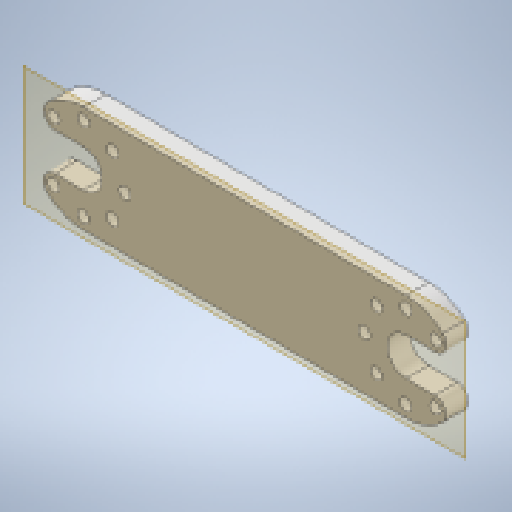
# Autodesk Inventor part: calf
Saved by Autodesk Inventor 2024 (Build 280153000, 153)
## iProperties
Created: 2024-09-17
Part Number: calf
Material: PMMA 플라스틱
Document SubType Name: Modeling
Designer: Eungang
Density: 1.188 g/cm^3
Appearance: 폴리카보네이트 - 선명
Author: Eungang
Autodesk Inventor part; units mm, degrees
ref_plane "YZ Plane" through (0, 0, 0) normal (1, 0, 0) x (0, 1, 0)
ref_plane "XZ Plane" through (0, 0, 0) normal (0, 1, 0) x (-1, 0, 0)
ref_plane "XY Plane" through (0, 0, 0) normal (0, 0, 1) x (1, 0, 0)
ref_plane "작업 평면1" through (0, 0, 0) normal (0, 0, 1) x (1, 0, 0)
sketch "스케치1" plane through (0, 0, 0) normal (0, 0, 1) x (1, 0, 0)
  circle A0 centre (-5.2751, -1.5499) radius 1.55 projected
  circle A1 centre (2.5198, 1.6312) radius 1.55 projected
  circle A2 centre (-16.2175, 9.5075) radius 1.55 projected
  circle A3 centre (-13.0363, 1.7126) radius 1.55 projected
  circle A4 centre (-12.955, 17.2687) radius 1.55 projected
  circle A5 centre (-90.374, -1.1049) radius 1.55 projected
  circle A6 centre (-98.1352, 2.1575) radius 1.55 projected
  circle A7 centre (-79.3166, 9.8374) radius 1.55 projected
  circle A8 centre (-82.4977, 17.6323) radius 1.55 projected
  circle A9 centre (-82.579, 2.0762) radius 1.55 projected
  circle A10 centre (-98.0538, 17.7137) radius 1.55 projected
  circle A11 centre (-90.2589, 20.8948) radius 1.55 projected
  circle A12 centre (2.6011, 17.1874) radius 1.55 projected
  circle A13 centre (-5.1601, 20.4498) radius 1.55 projected
  arc A14 (4.3379, -0.782) -> (2.306, 4.4106) centre (2.2903, 1.4106) ccw projected
  line L0 (2.306, 4.4106) -> (-5.2438, 4.45) projected
  arc A15 (-5.1915, 14.4499) -> (-5.2438, 4.45) centre (-5.2176, 9.45) ccw projected
  line L1 (-5.1915, 14.4499) -> (2.3583, 14.4104) projected
  arc A16 (2.3583, 14.4104) -> (4.4444, 19.5814) centre (2.374, 17.4104) ccw projected
  arc A17 (4.4444, 19.5814) -> (-5.1444, 23.4498) centre (-5.2176, 9.45) ccw projected
  line L2 (-5.1444, 23.4498) -> (-90.2432, 23.8948) projected
  arc A18 (-90.2432, 23.8948) -> (-99.872, 20.1269) centre (-90.3164, 9.8949) ccw projected
  arc A19 (-99.872, 20.1269) -> (-97.84, 14.9344) centre (-97.8243, 17.9343) ccw projected
  line L3 (-97.84, 14.9344) -> (-90.2903, 14.8949) projected
  arc A20 (-90.3426, 4.895) -> (-90.2903, 14.8949) centre (-90.3164, 9.8949) ccw projected
  line L4 (-90.3426, 4.895) -> (-97.8923, 4.9345) projected
  arc A21 (-97.8923, 4.9345) -> (-99.9784, -0.2365) centre (-97.908, 1.9345) ccw projected
  arc A22 (-99.9784, -0.2365) -> (-90.3897, -4.1049) centre (-90.3164, 9.8949) ccw projected
  line L5 (-90.3897, -4.1049) -> (-90.3897, -4.1065) projected
  line L6 (-90.3897, -4.1065) -> (-5.2908, -4.5515) projected
  line L7 (-5.2908, -4.5515) -> (-5.2908, -4.5498) projected
  arc A23 (-5.2908, -4.5498) -> (4.3379, -0.782) centre (-5.2176, 9.45) ccw projected
  circle A24 centre (-5.2176, 9.45) radius 1.5 projected
  circle A25 centre (-5.2176, 9.45) radius 5.2
  line L8 (-5.2176, 4.25) -> (6.1788, 4.25)
  line L9 (6.1788, 4.25) -> (6.1788, 14.65)
  line L10 (6.1788, 14.65) -> (-5.2176, 14.65)
  line L11 (-5.2176, 14.65) -> (-5.2176, 4.25)
  circle A26 centre (-12.955, 17.2687) radius 1.35
  circle A27 centre (-16.2175, 9.5075) radius 1.35
  circle A28 centre (-13.0363, 1.7126) radius 1.35
  circle A29 centre (-5.2751, -1.5499) radius 1.35
  circle A30 centre (2.5198, 1.6312) radius 1.35
  circle A31 centre (5.7822, 9.3924) radius 1.35
  circle A32 centre (2.6011, 17.1874) radius 1.35
  circle A33 centre (-5.1601, 20.4498) radius 1.35
  line L12 (-47.6938, 23.6723) -> (-47.8402, -4.329)
  circle A34 centre (-90.374, -1.1049) radius 1.55
  circle A35 centre (-98.1352, 2.1575) radius 1.55
  circle A36 centre (-79.3166, 9.8374) radius 1.55
  circle A37 centre (-82.579, 2.0762) radius 1.55
  circle A38 centre (-82.4977, 17.6323) radius 1.55
  circle A39 centre (-98.0538, 17.7137) radius 1.55
  circle A40 centre (-90.2589, 20.8948) radius 1.55
  arc A41 (-97.8923, 4.9345) -> (-99.9784, -0.2365) centre (-97.908, 1.9345) ccw
  line L13 (-97.8923, 4.9345) -> (-90.3426, 4.895)
  arc A42 (-90.3426, 4.895) -> (-90.2903, 14.8949) centre (-90.3164, 9.8949) ccw
  line L14 (-90.2903, 14.8949) -> (-97.84, 14.9344)
  arc A43 (-99.872, 20.1269) -> (-97.84, 14.9344) centre (-97.8243, 17.9343) ccw
  arc A44 (-90.2432, 23.8948) -> (-99.872, 20.1269) centre (-90.3164, 9.8949) ccw
  line L15 (-90.3897, -4.1065) -> (-90.3897, -4.1049)
  arc A45 (-99.9784, -0.2365) -> (-90.3897, -4.1049) centre (-90.3164, 9.8949) ccw
  circle A46 centre (-90.3164, 9.8949) radius 1.5
  circle A47 centre (-90.3164, 9.8949) radius 5.2
  line L16 (-90.3708, 4.6952) -> (-101.7666, 4.8144)
  line L17 (-101.7666, 4.8144) -> (-101.6578, 15.2138)
  line L18 (-101.6578, 15.2138) -> (-90.2621, 15.0947)
  line L19 (-90.2621, 15.0947) -> (-90.3708, 4.6952)
  circle A48 centre (-82.4977, 17.6323) radius 1.35
  circle A49 centre (-79.3166, 9.8374) radius 1.35
  circle A50 centre (-82.579, 2.0762) radius 1.35
  circle A51 centre (-90.374, -1.1049) radius 1.35
  circle A52 centre (-98.1352, 2.1575) radius 1.35
  circle A53 centre (-101.3163, 9.9525) radius 1.35
  circle A54 centre (-98.0538, 17.7137) radius 1.35
  circle A55 centre (-90.2589, 20.8948) radius 1.35
  point P0 (3.2588, 4.25)
  point P1 (-5.2176, 14.65)
  point P2 (3.5487, 14.65)
  point P3 (-99.0279, 15.1863)
  point P4 (-98.8468, 4.7839)
  dimension "d3" = 0.2
  dimension "d6" = 360
  constraints: 29 centre point, 25 symmetric about line, 24 end point, 10 point on circle, 2 midpoint, 2 parallel, 1 horizontal, 1 perpendicular, 45 other
  measures "d3" radial gap between concentric circles of A4 A26
extrude "돌출1" add sketch "스케치1" against normal blind 6 contours A0 | A1 | A2 | A3 | A4 | A5 | A6 | A7 | A8 | A9 | A10 | A11 | A12 | A13 | A23 L6 L12 L2 A17 A16 L10 A25 L8 A14 | L6 A22 A21 L16 A47 L18 A19 A18 L2 L12
